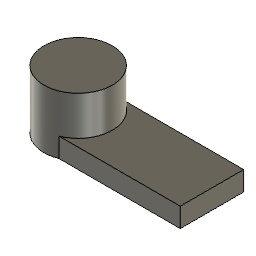
WiFi_Controlled_Desk_Lamp_Button (Autodesk Fusion 360 design; units mm, degrees)
part number: 2026-05-21-09-30-18-419
Autodesk Fusion 360 part; units mm, degrees
sketch "Sketch1" plane through (0, 0, 0) normal (0, 0, 1) x (1, 0, 0)
  circle A0 centre (0, 0) radius 3.5
  dimension "d1" = 7
  constraint coincident A0.centre origin
  measures "d1" diameter of A0
extrude "Extrude1" add sketch "Sketch1" along normal blind 6
sketch "Sketch2" plane through (0, 0, 0) normal (0, 0, 1) x (1, 0, 0)
  line L0 (0, 3.25) -> (13.701, 3.25)
  line L1 (13.701, 3.25) -> (13.701, -3.25)
  line L2 (13.701, -3.25) -> (0, -3.25)
  line L3 (0, -3.25) -> (0, 3.25)
  dimension "d4" = 6.5
  dimension "d5" = 13.701
  constraint horizontal L0
  constraint vertical L1
  constraint horizontal L2
  constraint vertical L3
  constraint midpoint origin L3
  measures "d4" distance of L0.start L2.end
  measures "d5" distance of L1.end L2.end
extrude "Extrude2" add sketch "Sketch2" along normal blind 2
